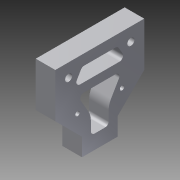
# Autodesk Inventor part: Arm_MiniLink_1
Saved by Autodesk Inventor 2013 (Build 170138000, 138)
## iProperties
Created: 2014-05-16
Part Number: Arm_MiniLink_1
Material: アセタール樹脂、白
Document SubType Name: Modeling
Designer: andou
Density: 1.425 g/cm^3
Mass: 22.1922 g
Surface Area: 69.6731 cm^2
Volume: 15.5734 cm^3
Author: andou
Autodesk Inventor part; units mm, degrees
ref_plane "YZ Plane" through (0, 0, 0) normal (1, 0, 0) x (0, 1, 0)
ref_plane "XZ Plane" through (0, 0, 0) normal (0, 1, 0) x (-1, 0, 0)
ref_plane "XY Plane" through (0, 0, 0) normal (0, 0, 1) x (1, 0, 0)
sketch "スケッチ1" plane through (0, 0, 0) normal (1, 0, 0) x (0, 1, 0)
  line L0 (50, 50) -> (-50, 50)
  line L1 (-50, 50) -> (-50, -50)
  line L2 (-50, -50) -> (50, -50)
  line L3 (50, -50) -> (50, 50)
  point P0 (0, 0)
  dimension "d0" = 100
  dimension "d2" = 100
  dimension "d3" = 50
  dimension "d4" = 50
  constraints: 8 end point, 2 parallel, 1 horizontal, 1 perpendicular
  measures "d0" distance of L1.end L2.end
  measures "d2" distance of L0.end L1.end
  measures "d3" distance from line of point (0, 0) L0
  measures "d4" distance from line of L1 point (0, 0)
extrude "押し出し1" add sketch "スケッチ1" along normal blind 11
sketch "スケッチ2" plane through (11, 0, 0) normal (1, 0, 0) x (0, 0, -1)
  line L0 (-50, 50) -> (-50, -50) projected
  line L1 (-50, -50) -> (50, -50) projected
  line L2 (50, -50) -> (50, 50) projected
  line L3 (50, 50) -> (-50, 50) projected
  line L4 (-25, -50) -> (-10, -35)
  line L5 (-10, -35) -> (15, -35)
  line L6 (15, -35) -> (50, -25.6218)
  line L7 (-50, 0) -> (-25, 0)
  line L8 (-25, 0) -> (-10, -15)
  line L9 (-10, -15) -> (12.367, -15)
  line L10 (12.367, -15) -> (30, -10.2752)
  line L11 (30, -10.2752) -> (30, 50)
  line L12 (-25, -50) -> (-50, -50)
  line L13 (-50, -50) -> (-50, 0)
  point P0 (0, 0)
  dimension "d7" = 135
  dimension "d8" = 135
  dimension "d9" = 25
  dimension "d10" = 25
  dimension "d11" = 50
  dimension "d16" = 165
  dimension "d17" = 20
  dimension "d18" = 20
  dimension "d89" = 20
  dimension "d90" = 25
  constraints: 20 end point, 4 parallel, 3 point on line, 2 collinear, 2 perpendicular, 1 midpoint
  measures "d7" angle of L1 L4
  measures "d8" angle of L8 L9
  measures "d9" distance of L4.start L0.end
  measures "d10" distance of L7.start L7.end
  measures "d11" distance between parallel lines of L1 L7
  measures "d16" angle of L6 L5
  measures "d17" distance between parallel lines of L2 L11
  measures "d18" distance between parallel lines of L6 L10
  measures "d89" distance between parallel lines of L9 L5
  measures "d90" distance of L4.end L5.end
extrude "押し出し2" cut sketch "スケッチ2" against normal blind 11 contours L7 L8 L9 L10 L11 L3 L2 L6 L5 L4 L1 L0 keep common part
sketch "スケッチ3" plane through (11, 0, 0) normal (1, 0, 0) x (0, 0, -1)
  line L0 (30, -10.2752) -> (30, 50) projected
  line L1 (12.367, -15) -> (30, -10.2752) projected
  line L2 (-10, -15) -> (12.367, -15) projected
  line L3 (-25, 0) -> (-10, -15) projected
  line L4 (-50, 0) -> (-25, 0) projected
  line L5 (-50, 0) -> (-50, -50) projected
  line L6 (-50, -50) -> (-25, -50) projected
  line L7 (-10, -35) -> (-25, -50) projected
  line L8 (15, -35) -> (-10, -35) projected
  line L9 (50, -25.6218) -> (15, -35) projected
  line L10 (50, -25.6218) -> (50, 50) projected
  line L11 (50, 50) -> (30, 50) projected
  circle A0 centre (-42.5, -7.5) radius 2
  circle A1 centre (-42.5, -42.5) radius 2
  circle A2 centre (-22.5, -12.5) radius 1.25
  circle A3 centre (-22.5, -37.5) radius 1.25
  arc A4 (36, 46) -> (44, 46) centre (40, 46) ccw
  line L12 (36, 46) -> (36, 50)
  line L13 (44, 46) -> (44, 50)
  point P0 (0, 0)
  dimension "d21" = 8
  dimension "d25" = 4
  dimension "d30" = 6
  dimension "d31" = 4
  dimension "d35" = 25
  dimension "d36" = 35
  dimension "d37" = 12.5
  dimension "d38" = 7.5
  dimension "d40" = 7.5
  dimension "d41" = 7.5
  dimension "d61" = 2.5
  dimension "d68" = 20
  dimension "d69" = 20
  constraints: 5 centre point, 4 end point, 2 equal radius, 2 perpendicular, 2 point on circle, 2 point on line, 2 tangent
  measures "d21" diameter of A4
  measures "d25" diameter of A0
  measures "d30" distance between parallel lines of L0 L12
  measures "d31" distance from line of L11 A4.centre
  measures "d35" distance of A3.centre A2.centre
  measures "d36" distance of A0.centre A1.centre
  measures "d37" distance from line of A3.centre L6
  measures "d38" distance from line of L6 A1.centre
  measures "d40" distance from line of A1.centre L5
  measures "d41" distance from line of L5 A0.centre
  measures "d61" diameter of A2
  measures "d68" horizontal distance of A0.centre A2.centre
  measures "d69" horizontal distance of A3.centre A1.centre
extrude "押し出し5" cut sketch "スケッチ3" against normal blind 11 contours L0 L11 L12 A4 L13 L10 L9 L8 L7 L6 L5 L4 L3 L2 L1 keep common part
sketch "スケッチ4" plane through (11, 0, 0) normal (1, 0, 0) x (0, 0, -1)
  line L0 (50, 50) -> (30, 50) projected
  circle A0 centre (33, 46) radius 1
  arc A1 (36, 46) -> (44, 46) centre (40, 46) ccw projected
  point P0 (0, 0)
  dimension "d47" = 4
  dimension "d49" = 2
  dimension "d64" = 7
  constraints: 1 centre point
  measures "d47" distance from line of L0 A0.centre
  measures "d49" diameter of A0
  measures "d64" distance of A1.centre A0.centre
hole "穴1" at (11, 46, -33) direction (-1, 0, 0) diameter 2 end through all
pattern_circular "円形状パターン2" count 5 over 180 about axis through (11, 46, -40) along (1, 0, 0) of "穴1"
sketch "スケッチ5" plane through (11, 0, 0) normal (1, 0, 0) x (0, 0, -1)
  line L0 (-10, -15) -> (12.367, -15) projected
  circle A0 centre (-22.5, -12.5) radius 1.25 projected
  circle A1 centre (-22.5, -37.5) radius 1.25 projected
  circle A2 centre (2.5, -20) radius 1.3
  circle A3 centre (2.5, -30) radius 1.3
  point P0 (0, 0)
  dimension "d70" = 2.6
  dimension "d74" = 5
  dimension "d75" = 10
  dimension "d91" = 25
  dimension "d92" = 25
  constraints: 2 centre point, 1 equal radius
  measures "d70" diameter of A3
  measures "d74" distance from line of L0 A2.centre
  measures "d75" distance of A2.centre A3.centre
  measures "d91" horizontal distance of A2.centre A0.centre
  measures "d92" horizontal distance of A1.centre A3.centre
hole "穴2" at (11, -20, -2.5) at (11, -30, -2.5) direction (-1, 0, 0) diameter 2.2 end through all
sketch "スケッチ6" plane through (11, 0, 0) normal (1, 0, 0) x (0, 0, -1)
  circle A0 centre (2.5, -20) radius 1.1 projected
  circle A1 centre (2.5, -30) radius 1.1 projected
  line L0 (12.367, -15) -> (30, -10.2752) projected
  line L1 (-10, -15) -> (12.367, -15) projected
  line L2 (-25, 0) -> (-10, -15) projected
  line L3 (-50, 0) -> (-25, 0) projected
  line L4 (-50, 0) -> (-50, -50) projected
  line L5 (-50, -50) -> (-25, -50) projected
  line L6 (-10, -35) -> (-25, -50) projected
  line L7 (15, -35) -> (-10, -35) projected
  line L8 (50, -25.6218) -> (15, -35) projected
  circle A2 centre (-22.5, -12.5) radius 1.25 projected
  circle A3 centre (-22.5, -37.5) radius 1.25 projected
  circle A4 centre (-42.5, -7.5) radius 2 projected
  circle A5 centre (-42.5, -42.5) radius 2 projected
  line L9 (0, -15) -> (0, -35)
  point P0 (0, 0)
  dimension "d93" = 10
  constraints: 2 end point, 2 point on line, 1 perpendicular
  measures "d93" distance from line of L1.start L9
extrude "押し出し6" cut sketch "スケッチ6" against normal blind 11 contours L1 L9 L7 L6 L5 L4 L3 L2 keep common part
sketch "スケッチ7" plane through (11, 0, 0) normal (1, 0, 0) x (0, 0, -1)
  line L0 (-10, -15) -> (0, -15) projected
  line L1 (-50, 0) -> (-50, -50) projected
  line L2 (-50, -50) -> (-25, -50) projected
  line L3 (-31, -12.5) -> (-31, -37.5)
  line L4 (-31, -37.5) -> (-18.0096, -30)
  line L5 (-31, -12.5) -> (-18.0096, -20)
  line L6 (-18.0096, -20) -> (-8.0096, -20)
  line L7 (-8.0096, -20) -> (-8.0096, -30)
  line L8 (-8.0096, -30) -> (-18.0096, -30)
  circle A0 centre (-42.5, -42.5) radius 2 projected
  circle A1 centre (-42.5, -7.5) radius 2 projected
  circle A2 centre (-22.5, -37.5) radius 1.25 projected
  circle A3 centre (-22.5, -12.5) radius 1.25 projected
  line L9 (0, -15) -> (0, -35) projected
  line L10 (-25, 0) -> (-10, -15) projected
  line L11 (-50, 0) -> (-25, 0) projected
  line L12 (-10, -35) -> (-25, -50) projected
  line L13 (0, -35) -> (-10, -35) projected
  point P0 (0, 0)
  dimension "d101" = 25
  dimension "d102" = 12.5
  dimension "d105" = 150
  dimension "d106" = 150
  dimension "d107" = 10
  dimension "d109" = 10
  dimension "d110" = 5
  dimension "d120" = 19
  constraints: 12 end point, 1 parallel, 1 perpendicular
  measures "d101" distance of L3.start L3.end
  measures "d102" distance from line of L2 L3.end
  measures "d105" angle of L4 L8
  measures "d106" angle of L5 L6
  measures "d107" distance of L5.end L6.end
  measures "d109" distance between parallel lines of L8 L6
  measures "d110" distance between parallel lines of L0 L6
  measures "d120" distance between parallel lines of L1 L3
sketch "スケッチ8" plane through (11, 0, 0) normal (1, 0, 0) x (0, 0, -1)
  line L0 (0, -15) -> (0, -35) projected
  line L1 (-50, 0) -> (-25, 0) projected
  line L2 (0, -35) -> (-10, -35) projected
  line L3 (-36, -10.3812) -> (-36, -39.6188)
  line L4 (-36, -39.6188) -> (-44, -35)
  line L5 (-44, -35) -> (-44, -15)
  line L6 (-44, -15) -> (-36, -10.3812)
  point P0 (0, 0)
  dimension "d113" = 20
  dimension "d115" = 8
  dimension "d116" = 120
  dimension "d117" = 120
  dimension "d118" = 15
  dimension "d119" = 36
  constraints: 8 end point, 1 parallel, 1 perpendicular
  measures "d113" distance of L4.end L5.end
  measures "d115" horizontal distance of L5.end L3.start
  measures "d116" angle of L5 L6
  measures "d117" angle of L5 L4
  measures "d118" distance from line of L1 L5.end
  measures "d119" distance between parallel lines of L0 L3
extrude "押し出し11" cut sketch "スケッチ7" against normal blind 11 keep common part
extrude "押し出し12" cut sketch "スケッチ8" against normal blind 11
fillet "フィレット1" radius 10 2 edges at (5.5, -20, 18.0096) (5.5, -30, 18.0096)
fillet "フィレット2" radius 2 8 edges at (5.5, -12.5, 31) (5.5, -37.5, 31) (5.5, -35, 44) (5.5, -15, 44) (5.5, -10.3812, 36) (5.5, -39.6188, 36) (5.5, -30, 8.0096) (5.5, -20, 8.0096)
